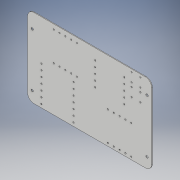
# Autodesk Inventor part: circuit board correct
Saved by Autodesk Inventor 2017 (Build 210142000, 142)
## iProperties
Created: 2017-06-14
Part Number: circuit board correct
Material: Generic
Document SubType Name: Modeling
Designer: slong
Density: 1 g/cm^3
Appearance: Default
Author: slong
Autodesk Inventor part; units mm, degrees
(part 1 of 2)
ref_plane "YZ Plane" through (0, 0, 0) normal (1, 0, 0) x (0, 1, 0)
ref_plane "XZ Plane" through (0, 0, 0) normal (0, 1, 0) x (-1, 0, 0)
ref_plane "XY Plane" through (0, 0, 0) normal (0, 0, 1) x (1, 0, 0)
sketch "Sketch1" plane through (0, 0, 0) normal (0, 0, 1) x (1, 0, 0)
  line L0 (17.0785, 215.8869) -> (322.9005, 215.8869)
  spline S0 degree 3 poles (322.9005, 215.8869) (332.3255, 215.8869) (339.9659, 208.2464) (339.9659, 198.8215) knots 1 1 1 1 2 2 2 2
  line L1 (322.9005, 215.8869) -> (332.3255, 215.8869) construction
  line L2 (332.3255, 215.8869) -> (339.9659, 208.2464) construction
  line L3 (339.9659, 208.2464) -> (339.9659, 198.8215) construction
  line L4 (339.9659, 198.8215) -> (339.9659, 17.0785)
  spline S1 degree 3 poles (339.9659, 17.0785) (339.9659, 7.6536) (332.3255, 0.0131) (322.9005, 0.0131) knots 3 3 3 3 4 4 4 4
  line L5 (339.9659, 17.0785) -> (339.9659, 7.6536) construction
  line L6 (339.9659, 7.6536) -> (332.3255, 0.0131) construction
  line L7 (332.3255, 0.0131) -> (322.9005, 0.0131) construction
  line L8 (322.9005, 0.0131) -> (17.0785, 0.0131)
  spline S2 degree 3 poles (17.0785, 0.0131) (7.6536, 0.0131) (0.0131, 7.6536) (0.0131, 17.0785) knots 5 5 5 5 6 6 6 6
  line L9 (17.0785, 0.0131) -> (7.6536, 0.0131) construction
  line L10 (7.6536, 0.0131) -> (0.0131, 7.6536) construction
  line L11 (0.0131, 7.6536) -> (0.0131, 17.0785) construction
  line L12 (0.0131, 17.0785) -> (0.0131, 198.8215)
  spline S3 degree 3 poles (0.0131, 198.8215) (0.0131, 208.2464) (7.6536, 215.8869) (17.0785, 215.8869) knots 7 7 7 7 8 8 8 8
  line L13 (0.0131, 198.8215) -> (0.0131, 208.2464) construction
  line L14 (0.0131, 208.2464) -> (7.6536, 215.8869) construction
  line L15 (7.6536, 215.8869) -> (17.0785, 215.8869) construction
  spline S4 degree 3 poles (12.7, 177.7884) (14.4471, 177.7884) (15.8634, 176.3721) (15.8634, 174.625) (15.8634, 172.8779) (14.4471, 171.4616) (12.7, 171.4616) (10.9529, 171.4616) (9.5366, 172.8779) (9.5366, 174.625) (9.5366, 176.3721) (10.9529, 177.7884) (12.7, 177.7884) knots 0 0 0 0 1 1 1 2 2 2 3 3 3 4 4 4 4
  line L16 (12.7, 177.7884) -> (14.4471, 177.7884) construction
  line L17 (14.4471, 177.7884) -> (15.8634, 176.3721) construction
  line L18 (15.8634, 176.3721) -> (15.8634, 174.625) construction
  line L19 (15.8634, 174.625) -> (15.8634, 172.8779) construction
  line L20 (15.8634, 172.8779) -> (14.4471, 171.4616) construction
  line L21 (14.4471, 171.4616) -> (12.7, 171.4616) construction
  line L22 (12.7, 171.4616) -> (10.9529, 171.4616) construction
  line L23 (10.9529, 171.4616) -> (9.5366, 172.8779) construction
  line L24 (9.5366, 172.8779) -> (9.5366, 174.625) construction
  line L25 (9.5366, 174.625) -> (9.5366, 176.3721) construction
  line L26 (9.5366, 176.3721) -> (10.9529, 177.7884) construction
  line L27 (10.9529, 177.7884) -> (12.7, 177.7884) construction
  spline S5 degree 3 poles (12.7, 31.7384) (14.4471, 31.7384) (15.8634, 30.3221) (15.8634, 28.575) (15.8634, 26.8279) (14.4471, 25.4116) (12.7, 25.4116) (10.9529, 25.4116) (9.5366, 26.8279) (9.5366, 28.575) (9.5366, 30.3221) (10.9529, 31.7384) (12.7, 31.7384) knots 0 0 0 0 1 1 1 2 2 2 3 3 3 4 4 4 4
  line L28 (12.7, 31.7384) -> (14.4471, 31.7384) construction
  line L29 (14.4471, 31.7384) -> (15.8634, 30.3221) construction
  line L30 (15.8634, 30.3221) -> (15.8634, 28.575) construction
  line L31 (15.8634, 28.575) -> (15.8634, 26.8279) construction
  line L32 (15.8634, 26.8279) -> (14.4471, 25.4116) construction
  line L33 (14.4471, 25.4116) -> (12.7, 25.4116) construction
  line L34 (12.7, 25.4116) -> (10.9529, 25.4116) construction
  line L35 (10.9529, 25.4116) -> (9.5366, 26.8279) construction
  line L36 (9.5366, 26.8279) -> (9.5366, 28.575) construction
  line L37 (9.5366, 28.575) -> (9.5366, 30.3221) construction
  line L38 (9.5366, 30.3221) -> (10.9529, 31.7384) construction
  line L39 (10.9529, 31.7384) -> (12.7, 31.7384) construction
  spline S6 degree 3 poles (327.279, 177.7884) (329.0261, 177.7884) (330.4424, 176.3721) (330.4424, 174.625) (330.4424, 172.8779) (329.0261, 171.4616) (327.279, 171.4616) (325.5319, 171.4616) (324.1156, 172.8779) (324.1156, 174.625) (324.1156, 176.3721) (325.5319, 177.7884) (327.279, 177.7884) knots 0 0 0 0 1 1 1 2 2 2 3 3 3 4 4 4 4
  line L40 (327.279, 177.7884) -> (329.0261, 177.7884) construction
  line L41 (329.0261, 177.7884) -> (330.4424, 176.3721) construction
  line L42 (330.4424, 176.3721) -> (330.4424, 174.625) construction
  line L43 (330.4424, 174.625) -> (330.4424, 172.8779) construction
  line L44 (330.4424, 172.8779) -> (329.0261, 171.4616) construction
  line L45 (329.0261, 171.4616) -> (327.279, 171.4616) construction
  line L46 (327.279, 171.4616) -> (325.5319, 171.4616) construction
  line L47 (325.5319, 171.4616) -> (324.1156, 172.8779) construction
  line L48 (324.1156, 172.8779) -> (324.1156, 174.625) construction
  line L49 (324.1156, 174.625) -> (324.1156, 176.3721) construction
  line L50 (324.1156, 176.3721) -> (325.5319, 177.7884) construction
  line L51 (325.5319, 177.7884) -> (327.279, 177.7884) construction
  spline S7 degree 3 poles (327.279, 31.7384) (329.0261, 31.7384) (330.4424, 30.3221) (330.4424, 28.575) (330.4424, 26.8279) (329.0261, 25.4116) (327.279, 25.4116) (325.5319, 25.4116) (324.1156, 26.8279) (324.1156, 28.575) (324.1156, 30.3221) (325.5319, 31.7384) (327.279, 31.7384) knots 0 0 0 0 1 1 1 2 2 2 3 3 3 4 4 4 4
  line L52 (327.279, 31.7384) -> (329.0261, 31.7384) construction
  line L53 (329.0261, 31.7384) -> (330.4424, 30.3221) construction
  line L54 (330.4424, 30.3221) -> (330.4424, 28.575) construction
  line L55 (330.4424, 28.575) -> (330.4424, 26.8279) construction
  line L56 (330.4424, 26.8279) -> (329.0261, 25.4116) construction
  line L57 (329.0261, 25.4116) -> (327.279, 25.4116) construction
  line L58 (327.279, 25.4116) -> (325.5319, 25.4116) construction
  line L59 (325.5319, 25.4116) -> (324.1156, 26.8279) construction
  line L60 (324.1156, 26.8279) -> (324.1156, 28.575) construction
  line L61 (324.1156, 28.575) -> (324.1156, 30.3221) construction
  line L62 (324.1156, 30.3221) -> (325.5319, 31.7384) construction
  line L63 (325.5319, 31.7384) -> (327.279, 31.7384) construction
  spline S8 degree 3 poles (310.8612, 184.086) (310.8612, 183.106) (310.0414, 182.3108) (309.0314, 182.3108) (308.0224, 182.3108) (307.2012, 183.106) (307.2012, 184.086) (307.2012, 185.0656) (308.0224, 185.8608) (309.0314, 185.8608) (310.0414, 185.8608) (310.8612, 185.0656) (310.8612, 184.086) knots 0 0 0 0 1 1 1 2 2 2 3 3 3 4 4 4 4
  line L64 (310.8612, 184.086) -> (310.8612, 183.106) construction
  line L65 (310.8612, 183.106) -> (310.0414, 182.3108) construction
  line L66 (310.0414, 182.3108) -> (309.0314, 182.3108) construction
  line L67 (309.0314, 182.3108) -> (308.0224, 182.3108) construction
  line L68 (308.0224, 182.3108) -> (307.2012, 183.106) construction
  line L69 (307.2012, 183.106) -> (307.2012, 184.086) construction
  line L70 (307.2012, 184.086) -> (307.2012, 185.0656) construction
  line L71 (307.2012, 185.0656) -> (308.0224, 185.8608) construction
  line L72 (308.0224, 185.8608) -> (309.0314, 185.8608) construction
  line L73 (309.0314, 185.8608) -> (310.0414, 185.8608) construction
  line L74 (310.0414, 185.8608) -> (310.8612, 185.0656) construction
  line L75 (310.8612, 185.0656) -> (310.8612, 184.086) construction
  spline S9 degree 3 poles (286.8614, 184.28) (286.8614, 183.2852) (286.0415, 182.4777) (285.0312, 182.4777) (284.0212, 182.4777) (283.2013, 183.2852) (283.2013, 184.28) (283.2013, 185.2752) (284.0212, 186.0827) (285.0312, 186.0827) (286.0415, 186.0827) (286.8614, 185.2752) (286.8614, 184.28) knots 0 0 0 0 1 1 1 2 2 2 3 3 3 4 4 4 4
  line L76 (286.8614, 184.28) -> (286.8614, 183.2852) construction
  line L77 (286.8614, 183.2852) -> (286.0415, 182.4777) construction
  line L78 (286.0415, 182.4777) -> (285.0312, 182.4777) construction
  line L79 (285.0312, 182.4777) -> (284.0212, 182.4777) construction
  line L80 (284.0212, 182.4777) -> (283.2013, 183.2852) construction
  line L81 (283.2013, 183.2852) -> (283.2013, 184.28) construction
  line L82 (283.2013, 184.28) -> (283.2013, 185.2752) construction
  line L83 (283.2013, 185.2752) -> (284.0212, 186.0827) construction
  line L84 (284.0212, 186.0827) -> (285.0312, 186.0827) construction
  line L85 (285.0312, 186.0827) -> (286.0415, 186.0827) construction
  line L86 (286.0415, 186.0827) -> (286.8614, 185.2752) construction
  line L87 (286.8614, 185.2752) -> (286.8614, 184.28) construction
  spline S10 degree 3 poles (310.8612, 207.9729) (310.8612, 206.9929) (310.0414, 206.1977) (309.0314, 206.1977) (308.0224, 206.1977) (307.2012, 206.9929) (307.2012, 207.9729) (307.2012, 208.9526) (308.0224, 209.7492) (309.0314, 209.7492) (310.0414, 209.7492) (310.8612, 208.9526) (310.8612, 207.9729) knots 0 0 0 0 1 1 1 2 2 2 3 3 3 4 4 4 4
  line L88 (310.8612, 207.9729) -> (310.8612, 206.9929) construction
  line L89 (310.8612, 206.9929) -> (310.0414, 206.1977) construction
  line L90 (310.0414, 206.1977) -> (309.0314, 206.1977) construction
  line L91 (309.0314, 206.1977) -> (308.0224, 206.1977) construction
  line L92 (308.0224, 206.1977) -> (307.2012, 206.9929) construction
  line L93 (307.2012, 206.9929) -> (307.2012, 207.9729) construction
  line L94 (307.2012, 207.9729) -> (307.2012, 208.9526) construction
  line L95 (307.2012, 208.9526) -> (308.0224, 209.7492) construction
  line L96 (308.0224, 209.7492) -> (309.0314, 209.7492) construction
  line L97 (309.0314, 209.7492) -> (310.0414, 209.7492) construction
  line L98 (310.0414, 209.7492) -> (310.8612, 208.9526) construction
  line L99 (310.8612, 208.9526) -> (310.8612, 207.9729) construction
  spline S11 degree 3 poles (286.8614, 208.1683) (286.8614, 207.1735) (286.0415, 206.366) (285.0312, 206.366) (284.0212, 206.366) (283.2013, 207.1735) (283.2013, 208.1683) (283.2013, 209.1635) (284.0212, 209.9711) (285.0312, 209.9711) (286.0415, 209.9711) (286.8614, 209.1635) (286.8614, 208.1683) knots 0 0 0 0 1 1 1 2 2 2 3 3 3 4 4 4 4
  line L100 (286.8614, 208.1683) -> (286.8614, 207.1735) construction
  line L101 (286.8614, 207.1735) -> (286.0415, 206.366) construction
  line L102 (286.0415, 206.366) -> (285.0312, 206.366) construction
  line L103 (285.0312, 206.366) -> (284.0212, 206.366) construction
  line L104 (284.0212, 206.366) -> (283.2013, 207.1735) construction
  line L105 (283.2013, 207.1735) -> (283.2013, 208.1683) construction
  line L106 (283.2013, 208.1683) -> (283.2013, 209.1635) construction
  line L107 (283.2013, 209.1635) -> (284.0212, 209.9711) construction
  line L108 (284.0212, 209.9711) -> (285.0312, 209.9711) construction
  line L109 (285.0312, 209.9711) -> (286.0415, 209.9711) construction
  line L110 (286.0415, 209.9711) -> (286.8614, 209.1635) construction
  line L111 (286.8614, 209.1635) -> (286.8614, 208.1683) construction
  spline S12 degree 3 poles (310.8612, 148.7399) (310.8612, 147.7599) (310.0414, 146.9647) (309.0314, 146.9647) (308.0224, 146.9647) (307.2012, 147.7599) (307.2012, 148.7399) (307.2012, 149.7196) (308.0224, 150.5147) (309.0314, 150.5147) (310.0414, 150.5147) (310.8612, 149.7196) (310.8612, 148.7399) knots 0 0 0 0 1 1 1 2 2 2 3 3 3 4 4 4 4
  line L112 (310.8612, 148.7399) -> (310.8612, 147.7599) construction
  line L113 (310.8612, 147.7599) -> (310.0414, 146.9647) construction
  line L114 (310.0414, 146.9647) -> (309.0314, 146.9647) construction
  line L115 (309.0314, 146.9647) -> (308.0224, 146.9647) construction
  line L116 (308.0224, 146.9647) -> (307.2012, 147.7599) construction
  line L117 (307.2012, 147.7599) -> (307.2012, 148.7399) construction
  line L118 (307.2012, 148.7399) -> (307.2012, 149.7196) construction
  line L119 (307.2012, 149.7196) -> (308.0224, 150.5147) construction
  line L120 (308.0224, 150.5147) -> (309.0314, 150.5147) construction
  line L121 (309.0314, 150.5147) -> (310.0414, 150.5147) construction
  line L122 (310.0414, 150.5147) -> (310.8612, 149.7196) construction
  line L123 (310.8612, 149.7196) -> (310.8612, 148.7399) construction
  spline S13 degree 3 poles (286.8614, 148.9339) (286.8614, 147.9391) (286.0415, 147.1316) (285.0312, 147.1316) (284.0212, 147.1316) (283.2013, 147.9391) (283.2013, 148.9339) (283.2013, 149.9291) (284.0212, 150.7366) (285.0312, 150.7366) (286.0415, 150.7366) (286.8614, 149.9291) (286.8614, 148.9339) knots 0 0 0 0 1 1 1 2 2 2 3 3 3 4 4 4 4
  line L124 (286.8614, 148.9339) -> (286.8614, 147.9391) construction
  line L125 (286.8614, 147.9391) -> (286.0415, 147.1316) construction
  line L126 (286.0415, 147.1316) -> (285.0312, 147.1316) construction
  line L127 (285.0312, 147.1316) -> (284.0212, 147.1316) construction
  line L128 (284.0212, 147.1316) -> (283.2013, 147.9391) construction
  line L129 (283.2013, 147.9391) -> (283.2013, 148.9339) construction
  line L130 (283.2013, 148.9339) -> (283.2013, 149.9291) construction
  line L131 (283.2013, 149.9291) -> (284.0212, 150.7366) construction
  line L132 (284.0212, 150.7366) -> (285.0312, 150.7366) construction
  line L133 (285.0312, 150.7366) -> (286.0415, 150.7366) construction
  line L134 (286.0415, 150.7366) -> (286.8614, 149.9291) construction
  line L135 (286.8614, 149.9291) -> (286.8614, 148.9339) construction
  spline S14 degree 3 poles (310.8612, 172.6269) (310.8612, 171.6469) (310.0414, 170.8517) (309.0314, 170.8517) (308.0224, 170.8517) (307.2012, 171.6469) (307.2012, 172.6269) (307.2012, 173.6065) (308.0224, 174.4031) (309.0314, 174.4031) (310.0414, 174.4031) (310.8612, 173.6065) (310.8612, 172.6269) knots 0 0 0 0 1 1 1 2 2 2 3 3 3 4 4 4 4
  line L136 (310.8612, 172.6269) -> (310.8612, 171.6469) construction
  line L137 (310.8612, 171.6469) -> (310.0414, 170.8517) construction
  line L138 (310.0414, 170.8517) -> (309.0314, 170.8517) construction
  line L139 (309.0314, 170.8517) -> (308.0224, 170.8517) construction
  line L140 (308.0224, 170.8517) -> (307.2012, 171.6469) construction
  line L141 (307.2012, 171.6469) -> (307.2012, 172.6269) construction
  line L142 (307.2012, 172.6269) -> (307.2012, 173.6065) construction
  line L143 (307.2012, 173.6065) -> (308.0224, 174.4031) construction
  line L144 (308.0224, 174.4031) -> (309.0314, 174.4031) construction
  line L145 (309.0314, 174.4031) -> (310.0414, 174.4031) construction
  line L146 (310.0414, 174.4031) -> (310.8612, 173.6065) construction
  line L147 (310.8612, 173.6065) -> (310.8612, 172.6269) construction
  spline S15 degree 3 poles (286.8614, 172.8223) (286.8614, 171.8274) (286.0415, 171.0199) (285.0312, 171.0199) (284.0212, 171.0199) (283.2013, 171.8274) (283.2013, 172.8223) (283.2013, 173.8175) (284.0212, 174.625) (285.0312, 174.625) (286.0415, 174.625) (286.8614, 173.8175) (286.8614, 172.8223) knots 0 0 0 0 1 1 1 2 2 2 3 3 3 4 4 4 4
  line L148 (286.8614, 172.8223) -> (286.8614, 171.8274) construction
  line L149 (286.8614, 171.8274) -> (286.0415, 171.0199) construction
  line L150 (286.0415, 171.0199) -> (285.0312, 171.0199) construction
  line L151 (285.0312, 171.0199) -> (284.0212, 171.0199) construction
  line L152 (284.0212, 171.0199) -> (283.2013, 171.8274) construction
  line L153 (283.2013, 171.8274) -> (283.2013, 172.8223) construction
  line L154 (283.2013, 172.8223) -> (283.2013, 173.8175) construction
  line L155 (283.2013, 173.8175) -> (284.0212, 174.625) construction
  line L156 (284.0212, 174.625) -> (285.0312, 174.625) construction
  line L157 (285.0312, 174.625) -> (286.0415, 174.625) construction
  line L158 (286.0415, 174.625) -> (286.8614, 173.8175) construction
  line L159 (286.8614, 173.8175) -> (286.8614, 172.8223) construction
  spline S16 degree 3 poles (73.3234, 122.6835) (73.3234, 121.6731) (72.5036, 120.8533) (71.4936, 120.8533) (70.4832, 120.8533) (69.6634, 121.6731) (69.6634, 122.6835) (69.6634, 123.6935) (70.4832, 124.5134) (71.4936, 124.5134) (72.5036, 124.5134) (73.3234, 123.6935) (73.3234, 122.6835) knots 0 0 0 0 1 1 1 2 2 2 3 3 3 4 4 4 4
  line L160 (73.3234, 122.6835) -> (73.3234, 121.6731) construction
  line L161 (73.3234, 121.6731) -> (72.5036, 120.8533) construction
  line L162 (72.5036, 120.8533) -> (71.4936, 120.8533) construction
  line L163 (71.4936, 120.8533) -> (70.4832, 120.8533) construction
  line L164 (70.4832, 120.8533) -> (69.6634, 121.6731) construction
  line L165 (69.6634, 121.6731) -> (69.6634, 122.6835) construction
  line L166 (69.6634, 122.6835) -> (69.6634, 123.6935) construction
  line L167 (69.6634, 123.6935) -> (70.4832, 124.5134) construction
  line L168 (70.4832, 124.5134) -> (71.4936, 124.5134) construction
  line L169 (71.4936, 124.5134) -> (72.5036, 124.5134) construction
  line L170 (72.5036, 124.5134) -> (73.3234, 123.6935) construction
  line L171 (73.3234, 123.6935) -> (73.3234, 122.6835) construction
  spline S17 degree 3 poles (89.324, 122.6835) (89.324, 121.6731) (88.5038, 120.8533) (87.4938, 120.8533) (86.4838, 120.8533) (85.6639, 121.6731) (85.6639, 122.6835) (85.6639, 123.6935) (86.4838, 124.5134) (87.4938, 124.5134) (88.5038, 124.5134) (89.324, 123.6935) (89.324, 122.6835) knots 0 0 0 0 1 1 1 2 2 2 3 3 3 4 4 4 4
  line L172 (89.324, 122.6835) -> (89.324, 121.6731) construction
  line L173 (89.324, 121.6731) -> (88.5038, 120.8533) construction
  line L174 (88.5038, 120.8533) -> (87.4938, 120.8533) construction
  line L175 (87.4938, 120.8533) -> (86.4838, 120.8533) construction
  line L176 (86.4838, 120.8533) -> (85.6639, 121.6731) construction
  line L177 (85.6639, 121.6731) -> (85.6639, 122.6835) construction
  line L178 (85.6639, 122.6835) -> (85.6639, 123.6935) construction
  line L179 (85.6639, 123.6935) -> (86.4838, 124.5134) construction
  line L180 (86.4838, 124.5134) -> (87.4938, 124.5134) construction
  line L181 (87.4938, 124.5134) -> (88.5038, 124.5134) construction
  line L182 (88.5038, 124.5134) -> (89.324, 123.6935) construction
  line L183 (89.324, 123.6935) -> (89.324, 122.6835) construction
  spline S18 degree 3 poles (101.6656, 122.62) (101.6656, 121.6153) (102.4854, 120.7997) (103.4955, 120.7997) (104.5058, 120.7997) (105.3257, 121.6153) (105.3257, 122.62) (105.3257, 123.6247) (104.5058, 124.4417) (103.4955, 124.4417) (102.4854, 124.4417) (101.6656, 123.6247) (101.6656, 122.62) knots 0 0 0 0 1 1 1 2 2 2 3 3 3 4 4 4 4
  line L184 (101.6656, 122.62) -> (101.6656, 121.6153) construction
  line L185 (101.6656, 121.6153) -> (102.4854, 120.7997) construction
  line L186 (102.4854, 120.7997) -> (103.4955, 120.7997) construction
  line L187 (103.4955, 120.7997) -> (104.5058, 120.7997) construction
  line L188 (104.5058, 120.7997) -> (105.3257, 121.6153) construction
  line L189 (105.3257, 121.6153) -> (105.3257, 122.62) construction
  line L190 (105.3257, 122.62) -> (105.3257, 123.6247) construction
  line L191 (105.3257, 123.6247) -> (104.5058, 124.4417) construction
  line L192 (104.5058, 124.4417) -> (103.4955, 124.4417) construction
  line L193 (103.4955, 124.4417) -> (102.4854, 124.4417) construction
  line L194 (102.4854, 124.4417) -> (101.6656, 123.6247) construction
  line L195 (101.6656, 123.6247) -> (101.6656, 122.62) construction
  spline S19 degree 3 poles (121.3259, 122.62) (121.3259, 121.6153) (120.506, 120.7997) (119.496, 120.7997) (118.486, 120.7997) (117.6658, 121.6153) (117.6658, 122.62) (117.6658, 123.6247) (118.486, 124.4417) (119.496, 124.4417) (120.506, 124.4417) (121.3259, 123.6247) (121.3259, 122.62) knots 0 0 0 0 1 1 1 2 2 2 3 3 3 4 4 4 4
  line L196 (121.3259, 122.62) -> (121.3259, 121.6153) construction
  line L197 (121.3259, 121.6153) -> (120.506, 120.7997) construction
  line L198 (120.506, 120.7997) -> (119.496, 120.7997) construction
  line L199 (119.496, 120.7997) -> (118.486, 120.7997) construction
  line L200 (118.486, 120.7997) -> (117.6658, 121.6153) construction
  line L201 (117.6658, 121.6153) -> (117.6658, 122.62) construction
  line L202 (117.6658, 122.62) -> (117.6658, 123.6247) construction
  line L203 (117.6658, 123.6247) -> (118.486, 124.4417) construction
  line L204 (118.486, 124.4417) -> (119.496, 124.4417) construction
  line L205 (119.496, 124.4417) -> (120.506, 124.4417) construction
  line L206 (120.506, 124.4417) -> (121.3259, 123.6247) construction
  line L207 (121.3259, 123.6247) -> (121.3259, 122.62) construction
  spline S20 degree 3 poles (137.3265, 122.4905) (137.3265, 121.4953) (136.5052, 120.6878) (135.4963, 120.6878) (134.4863, 120.6878) (133.6664, 121.4953) (133.6664, 122.4905) (133.6664, 123.4854) (134.4863, 124.2929) (135.4963, 124.2929) (136.5052, 124.2929) (137.3265, 123.4854) (137.3265, 122.4905) knots 0 0 0 0 1 1 1 2 2 2 3 3 3 4 4 4 4
  line L208 (137.3265, 122.4905) -> (137.3265, 121.4953) construction
  line L209 (137.3265, 121.4953) -> (136.5052, 120.6878) construction
  line L210 (136.5052, 120.6878) -> (135.4963, 120.6878) construction
  line L211 (135.4963, 120.6878) -> (134.4863, 120.6878) construction
  line L212 (134.4863, 120.6878) -> (133.6664, 121.4953) construction
  line L213 (133.6664, 121.4953) -> (133.6664, 122.4905) construction
  line L214 (133.6664, 122.4905) -> (133.6664, 123.4854) construction
  line L215 (133.6664, 123.4854) -> (134.4863, 124.2929) construction
  line L216 (134.4863, 124.2929) -> (135.4963, 124.2929) construction
  line L217 (135.4963, 124.2929) -> (136.5052, 124.2929) construction
  line L218 (136.5052, 124.2929) -> (137.3265, 123.4854) construction
  line L219 (137.3265, 123.4854) -> (137.3265, 122.4905) construction
  spline S21 degree 3 poles (73.3236, 202.6826) (73.3236, 201.6726) (72.5034, 200.8527) (71.4934, 200.8527) (70.4834, 200.8527) (69.6636, 201.6726) (69.6636, 202.6826) (69.6636, 203.6926) (70.4834, 204.5128) (71.4934, 204.5128) (72.5034, 204.5128) (73.3236, 203.6926) (73.3236, 202.6826) knots 0 0 0 0 1 1 1 2 2 2 3 3 3 4 4 4 4
  line L220 (73.3236, 202.6826) -> (73.3236, 201.6726) construction
  line L221 (73.3236, 201.6726) -> (72.5034, 200.8527) construction
  line L222 (72.5034, 200.8527) -> (71.4934, 200.8527) construction
  line L223 (71.4934, 200.8527) -> (70.4834, 200.8527) construction
  line L224 (70.4834, 200.8527) -> (69.6636, 201.6726) construction
  line L225 (69.6636, 201.6726) -> (69.6636, 202.6826) construction
  line L226 (69.6636, 202.6826) -> (69.6636, 203.6926) construction
  line L227 (69.6636, 203.6926) -> (70.4834, 204.5128) construction
  line L228 (70.4834, 204.5128) -> (71.4934, 204.5128) construction
  line L229 (71.4934, 204.5128) -> (72.5034, 204.5128) construction
  line L230 (72.5034, 204.5128) -> (73.3236, 203.6926) construction
  line L231 (73.3236, 203.6926) -> (73.3236, 202.6826) construction
  spline S22 degree 3 poles (89.3238, 202.6826) (89.3238, 201.6726) (88.504, 200.8527) (87.494, 200.8527) (86.4836, 200.8527) (85.6638, 201.6726) (85.6638, 202.6826) (85.6638, 203.6926) (86.4836, 204.5128) (87.494, 204.5128) (88.504, 204.5128) (89.3238, 203.6926) (89.3238, 202.6826) knots 0 0 0 0 1 1 1 2 2 2 3 3 3 4 4 4 4
  line L232 (89.3238, 202.6826) -> (89.3238, 201.6726) construction
  line L233 (89.3238, 201.6726) -> (88.504, 200.8527) construction
  line L234 (88.504, 200.8527) -> (87.494, 200.8527) construction
  line L235 (87.494, 200.8527) -> (86.4836, 200.8527) construction
  line L236 (86.4836, 200.8527) -> (85.6638, 201.6726) construction
  line L237 (85.6638, 201.6726) -> (85.6638, 202.6826) construction
  line L238 (85.6638, 202.6826) -> (85.6638, 203.6926) construction
  line L239 (85.6638, 203.6926) -> (86.4836, 204.5128) construction
  line L240 (86.4836, 204.5128) -> (87.494, 204.5128) construction
  line L241 (87.494, 204.5128) -> (88.504, 204.5128) construction
  line L242 (88.504, 204.5128) -> (89.3238, 203.6926) construction
  line L243 (89.3238, 203.6926) -> (89.3238, 202.6826) construction
  spline S23 degree 3 poles (105.3258, 202.6191) (105.3258, 201.6147) (104.5056, 200.7987) (103.4956, 200.7987) (102.4856, 200.7987) (101.6658, 201.6147) (101.6658, 202.6191) (101.6658, 203.6252) (102.4856, 204.4412) (103.4956, 204.4412) (104.5056, 204.4412) (105.3258, 203.6252) (105.3258, 202.6191) knots 0 0 0 0 1 1 1 2 2 2 3 3 3 4 4 4 4
  line L244 (105.3258, 202.6191) -> (105.3258, 201.6147) construction
  line L245 (105.3258, 201.6147) -> (104.5056, 200.7987) construction
  line L246 (104.5056, 200.7987) -> (103.4956, 200.7987) construction
  line L247 (103.4956, 200.7987) -> (102.4856, 200.7987) construction
  line L248 (102.4856, 200.7987) -> (101.6658, 201.6147) construction
  line L249 (101.6658, 201.6147) -> (101.6658, 202.6191) construction
  line L250 (101.6658, 202.6191) -> (101.6658, 203.6252) construction
  line L251 (101.6658, 203.6252) -> (102.4856, 204.4412) construction
  line L252 (102.4856, 204.4412) -> (103.4956, 204.4412) construction
  line L253 (103.4956, 204.4412) -> (104.5056, 204.4412) construction
  line L254 (104.5056, 204.4412) -> (105.3258, 203.6252) construction
  line L255 (105.3258, 203.6252) -> (105.3258, 202.6191) construction
  spline S24 degree 3 poles (121.326, 202.6191) (121.326, 201.6147) (120.5062, 200.7987) (119.4962, 200.7987) (118.4858, 200.7987) (117.6659, 201.6147) (117.6659, 202.6191) (117.6659, 203.6252) (118.4858, 204.4412) (119.4962, 204.4412) (120.5062, 204.4412) (121.326, 203.6252) (121.326, 202.6191) knots 0 0 0 0 1 1 1 2 2 2 3 3 3 4 4 4 4
  line L256 (121.326, 202.6191) -> (121.326, 201.6147) construction
  line L257 (121.326, 201.6147) -> (120.5062, 200.7987) construction
  line L258 (120.5062, 200.7987) -> (119.4962, 200.7987) construction
  line L259 (119.4962, 200.7987) -> (118.4858, 200.7987) construction
  line L260 (118.4858, 200.7987) -> (117.6659, 201.6147) construction
  line L261 (117.6659, 201.6147) -> (117.6659, 202.6191) construction
  line L262 (117.6659, 202.6191) -> (117.6659, 203.6252) construction
  line L263 (117.6659, 203.6252) -> (118.4858, 204.4412) construction
  line L264 (118.4858, 204.4412) -> (119.4962, 204.4412) construction
  line L265 (119.4962, 204.4412) -> (120.5062, 204.4412) construction
  line L266 (120.5062, 204.4412) -> (121.326, 203.6252) construction
  line L267 (121.326, 203.6252) -> (121.326, 202.6191) construction
  spline S25 degree 3 poles (137.3252, 202.4896) (137.3252, 201.4948) (136.5053, 200.6872) (135.495, 200.6872) (134.4864, 200.6872) (133.6665, 201.4948) (133.6665, 202.4896) (133.6665, 203.4848) (134.4864, 204.2923) (135.495, 204.2923) (136.5053, 204.2923) (137.3252, 203.4848) (137.3252, 202.4896) knots 0 0 0 0 1 1 1 2 2 2 3 3 3 4 4 4 4
  line L268 (137.3252, 202.4896) -> (137.3252, 201.4948) construction
  line L269 (137.3252, 201.4948) -> (136.5053, 200.6872) construction
  line L270 (136.5053, 200.6872) -> (135.495, 200.6872) construction
  line L271 (135.495, 200.6872) -> (134.4864, 200.6872) construction
  line L272 (134.4864, 200.6872) -> (133.6665, 201.4948) construction
  line L273 (133.6665, 201.4948) -> (133.6665, 202.4896) construction
  line L274 (133.6665, 202.4896) -> (133.6665, 203.4848) construction
  line L275 (133.6665, 203.4848) -> (134.4864, 204.2923) construction
  line L276 (134.4864, 204.2923) -> (135.495, 204.2923) construction
  line L277 (135.495, 204.2923) -> (136.5053, 204.2923) construction
  line L278 (136.5053, 204.2923) -> (137.3252, 203.4848) construction
  line L279 (137.3252, 203.4848) -> (137.3252, 202.4896) construction
  spline S26 degree 3 poles (126.1694, 103.4986) (125.1594, 103.4986) (124.3396, 104.3184) (124.3396, 105.3288) (124.3396, 106.3388) (125.1594, 107.1586) (126.1694, 107.1586) (127.1798, 107.1586) (127.9996, 106.3388) (127.9996, 105.3288) (127.9996, 104.3184) (127.1798, 103.4986) (126.1694, 103.4986) knots 0 0 0 0 1 1 1 2 2 2 3 3 3 4 4 4 4
  line L280 (126.1694, 103.4986) -> (125.1594, 103.4986) construction
  line L281 (125.1594, 103.4986) -> (124.3396, 104.3184) construction
  line L282 (124.3396, 104.3184) -> (124.3396, 105.3288) construction
  line L283 (124.3396, 105.3288) -> (124.3396, 106.3388) construction
  line L284 (124.3396, 106.3388) -> (125.1594, 107.1586) construction
  line L285 (125.1594, 107.1586) -> (126.1694, 107.1586) construction
  line L286 (126.1694, 107.1586) -> (127.1798, 107.1586) construction
  line L287 (127.1798, 107.1586) -> (127.9996, 106.3388) construction
  line L288 (127.9996, 106.3388) -> (127.9996, 105.3288) construction
  line L289 (127.9996, 105.3288) -> (127.9996, 104.3184) construction
  line L290 (127.9996, 104.3184) -> (127.1798, 103.4986) construction
  line L291 (127.1798, 103.4986) -> (126.1694, 103.4986) construction
  spline S27 degree 3 poles (126.1694, 87.4997) (125.1594, 87.4997) (124.3396, 88.3196) (124.3396, 89.3282) (124.3396, 90.3382) (125.1594, 91.1584) (126.1694, 91.1584) (127.1798, 91.1584) (127.9996, 90.3382) (127.9996, 89.3282) (127.9996, 88.3196) (127.1798, 87.4997) (126.1694, 87.4997) knots 0 0 0 0 1 1 1 2 2 2 3 3 3 4 4 4 4
  line L292 (126.1694, 87.4997) -> (125.1594, 87.4997) construction
  line L293 (125.1594, 87.4997) -> (124.3396, 88.3196) construction
  line L294 (124.3396, 88.3196) -> (124.3396, 89.3282) construction
  line L295 (124.3396, 89.3282) -> (124.3396, 90.3382) construction
  line L296 (124.3396, 90.3382) -> (125.1594, 91.1584) construction
  line L297 (125.1594, 91.1584) -> (126.1694, 91.1584) construction
  line L298 (126.1694, 91.1584) -> (127.1798, 91.1584) construction
  line L299 (127.1798, 91.1584) -> (127.9996, 90.3382) construction
  line L300 (127.9996, 90.3382) -> (127.9996, 89.3282) construction
  line L301 (127.9996, 89.3282) -> (127.9996, 88.3196) construction
  line L302 (127.9996, 88.3196) -> (127.1798, 87.4997) construction
  line L303 (127.1798, 87.4997) -> (126.1694, 87.4997) construction
  spline S28 degree 3 poles (126.1063, 71.4963) (125.1016, 71.4963) (124.286, 72.3165) (124.286, 73.3265) (124.286, 74.3365) (125.1016, 75.1564) (126.1063, 75.1564) (127.1106, 75.1564) (127.9266, 74.3365) (127.9266, 73.3265) (127.9266, 72.3165) (127.1107, 71.4963) (126.1063, 71.4963) knots 0 0 0 0 1 1 1 2 2 2 3 3 3 4 4 4 4
  line L304 (126.1063, 71.4963) -> (125.1016, 71.4963) construction
  line L305 (125.1016, 71.4963) -> (124.286, 72.3165) construction
  line L306 (124.286, 72.3165) -> (124.286, 73.3265) construction
  line L307 (124.286, 73.3265) -> (124.286, 74.3365) construction
  line L308 (124.286, 74.3365) -> (125.1016, 75.1564) construction
  line L309 (125.1016, 75.1564) -> (126.1063, 75.1564) construction
  line L310 (126.1063, 75.1564) -> (127.1106, 75.1564) construction
  line L311 (127.1106, 75.1564) -> (127.9266, 74.3365) construction
  line L312 (127.9266, 74.3365) -> (127.9266, 73.3265) construction
  line L313 (127.9266, 73.3265) -> (127.9266, 72.3165) construction
  line L314 (127.9266, 72.3165) -> (127.1107, 71.4963) construction
  line L315 (127.1107, 71.4963) -> (126.1063, 71.4963) construction
  spline S29 degree 3 poles (126.1063, 55.4975) (125.1016, 55.4975) (124.286, 56.3174) (124.286, 57.3274) (124.286, 58.3377) (125.1016, 59.1576) (126.1063, 59.1576) (127.1106, 59.1576) (127.9266, 58.3377) (127.9266, 57.3274) (127.9266, 56.3174) (127.1107, 55.4975) (126.1063, 55.4975) knots 0 0 0 0 1 1 1 2 2 2 3 3 3 4 4 4 4
  line L316 (126.1063, 55.4975) -> (125.1016, 55.4975) construction
  line L317 (125.1016, 55.4975) -> (124.286, 56.3174) construction
  line L318 (124.286, 56.3174) -> (124.286, 57.3274) construction
  line L319 (124.286, 57.3274) -> (124.286, 58.3377) construction
  line L320 (124.286, 58.3377) -> (125.1016, 59.1576) construction
  line L321 (125.1016, 59.1576) -> (126.1063, 59.1576) construction
  line L322 (126.1063, 59.1576) -> (127.1106, 59.1576) construction
  line L323 (127.1106, 59.1576) -> (127.9266, 58.3377) construction
  line L324 (127.9266, 58.3377) -> (127.9266, 57.3274) construction
  line L325 (127.9266, 57.3274) -> (127.9266, 56.3174) construction
  line L326 (127.9266, 56.3174) -> (127.1107, 55.4975) construction
  line L327 (127.1107, 55.4975) -> (126.1063, 55.4975) construction
  spline S30 degree 3 poles (125.9768, 39.4969) (124.9816, 39.4969) (124.1741, 40.3171) (124.1741, 41.3271) (124.1741, 42.3371) (124.9816, 43.157) (125.9768, 43.157) (126.9717, 43.157) (127.7792, 42.3371) (127.7792, 41.3271) (127.7792, 40.3171) (126.9717, 39.4969) (125.9768, 39.4969) knots 0 0 0 0 1 1 1 2 2 2 3 3 3 4 4 4 4
  line L328 (125.9768, 39.4969) -> (124.9816, 39.4969) construction
  line L329 (124.9816, 39.4969) -> (124.1741, 40.3171) construction
  line L330 (124.1741, 40.3171) -> (124.1741, 41.3271) construction
  line L331 (124.1741, 41.3271) -> (124.1741, 42.3371) construction
  line L332 (124.1741, 42.3371) -> (124.9816, 43.157) construction
  line L333 (124.9816, 43.157) -> (125.9768, 43.157) construction
  line L334 (125.9768, 43.157) -> (126.9717, 43.157) construction
  line L335 (126.9717, 43.157) -> (127.7792, 42.3371) construction
  line L336 (127.7792, 42.3371) -> (127.7792, 41.3271) construction
  line L337 (127.7792, 41.3271) -> (127.7792, 40.3171) construction
  line L338 (127.7792, 40.3171) -> (126.9717, 39.4969) construction
  line L339 (126.9717, 39.4969) -> (125.9768, 39.4969) construction
  spline S31 degree 3 poles (125.9768, 23.4967) (124.9816, 23.4967) (124.1741, 24.3165) (124.1741, 25.3265) (124.1741, 26.3369) (124.9816, 27.1567) (125.9768, 27.1567) (126.9717, 27.1567) (127.7792, 26.3369) (127.7792, 25.3265) (127.7792, 24.3165) (126.9717, 23.4967) (125.9768, 23.4967) knots 0 0 0 0 1 1 1 2 2 2 3 3 3 4 4 4 4
  line L340 (125.9768, 23.4967) -> (124.9816, 23.4967) construction
  line L341 (124.9816, 23.4967) -> (124.1741, 24.3165) construction
  line L342 (124.1741, 24.3165) -> (124.1741, 25.3265) construction
  line L343 (124.1741, 25.3265) -> (124.1741, 26.3369) construction
  line L344 (124.1741, 26.3369) -> (124.9816, 27.1567) construction
  line L345 (124.9816, 27.1567) -> (125.9768, 27.1567) construction
  line L346 (125.9768, 27.1567) -> (126.9717, 27.1567) construction
  line L347 (126.9717, 27.1567) -> (127.7792, 26.3369) construction
  line L348 (127.7792, 26.3369) -> (127.7792, 25.3265) construction
  line L349 (127.7792, 25.3265) -> (127.7792, 24.3165) construction
  line L350 (127.7792, 24.3165) -> (126.9717, 23.4967) construction
  line L351 (126.9717, 23.4967) -> (125.9768, 23.4967) construction
  spline S32 degree 3 poles (125.781, 7.4961) (124.8014, 7.4961) (124.0062, 8.3163) (124.0062, 9.3263) (124.0062, 10.3363) (124.8014, 11.1562) (125.781, 11.1562) (126.7607, 11.1562) (127.5573, 10.3363) (127.5573, 9.3263) (127.5573, 8.3163) (126.7607, 7.4961) (125.781, 7.4961) knots 0 0 0 0 1 1 1 2 2 2 3 3 3 4 4 4 4
  line L352 (125.781, 7.4961) -> (124.8014, 7.4961) construction
  line L353 (124.8014, 7.4961) -> (124.0062, 8.3163) construction
  line L354 (124.0062, 8.3163) -> (124.0062, 9.3263) construction
  line L355 (124.0062, 9.3263) -> (124.0062, 10.3363) construction
  line L356 (124.0062, 10.3363) -> (124.8014, 11.1562) construction
  line L357 (124.8014, 11.1562) -> (125.781, 11.1562) construction
  line L358 (125.781, 11.1562) -> (126.7607, 11.1562) construction
  line L359 (126.7607, 11.1562) -> (127.5573, 10.3363) construction
  line L360 (127.5573, 10.3363) -> (127.5573, 9.3263) construction
  line L361 (127.5573, 9.3263) -> (127.5573, 8.3163) construction
  line L362 (127.5573, 8.3163) -> (126.7607, 7.4961) construction
  line L363 (126.7607, 7.4961) -> (125.781, 7.4961) construction
  spline S33 degree 3 poles (38.1694, 103.4986) (37.1594, 103.4986) (36.3395, 104.3184) (36.3395, 105.3288) (36.3395, 106.3388) (37.1594, 107.1586) (38.1694, 107.1586) (39.1794, 107.1586) (39.9996, 106.3388) (39.9996, 105.3288) (39.9996, 104.3184) (39.1794, 103.4986) (38.1694, 103.4986) knots 0 0 0 0 1 1 1 2 2 2 3 3 3 4 4 4 4
  line L364 (38.1694, 103.4986) -> (37.1594, 103.4986) construction
  line L365 (37.1594, 103.4986) -> (36.3395, 104.3184) construction
  line L366 (36.3395, 104.3184) -> (36.3395, 105.3288) construction
  line L367 (36.3395, 105.3288) -> (36.3395, 106.3388) construction
  line L368 (36.3395, 106.3388) -> (37.1594, 107.1586) construction
  line L369 (37.1594, 107.1586) -> (38.1694, 107.1586) construction
  line L370 (38.1694, 107.1586) -> (39.1794, 107.1586) construction
  line L371 (39.1794, 107.1586) -> (39.9996, 106.3388) construction
  line L372 (39.9996, 106.3388) -> (39.9996, 105.3288) construction
  line L373 (39.9996, 105.3288) -> (39.9996, 104.3184) construction
  line L374 (39.9996, 104.3184) -> (39.1794, 103.4986) construction
  line L375 (39.1794, 103.4986) -> (38.1694, 103.4986) construction
  spline S34 degree 3 poles (38.1694, 87.4997) (37.1594, 87.4997) (36.3395, 88.3196) (36.3395, 89.3282) (36.3395, 90.3382) (37.1594, 91.1584) (38.1694, 91.1584) (39.1794, 91.1584) (39.9996, 90.3382) (39.9996, 89.3282) (39.9996, 88.3196) (39.1794, 87.4997) (38.1694, 87.4997) knots 0 0 0 0 1 1 1 2 2 2 3 3 3 4 4 4 4
  line L376 (38.1694, 87.4997) -> (37.1594, 87.4997) construction
  line L377 (37.1594, 87.4997) -> (36.3395, 88.3196) construction
  line L378 (36.3395, 88.3196) -> (36.3395, 89.3282) construction
  line L379 (36.3395, 89.3282) -> (36.3395, 90.3382) construction
  line L380 (36.3395, 90.3382) -> (37.1594, 91.1584) construction
  line L381 (37.1594, 91.1584) -> (38.1694, 91.1584) construction
  line L382 (38.1694, 91.1584) -> (39.1794, 91.1584) construction
  line L383 (39.1794, 91.1584) -> (39.9996, 90.3382) construction
  line L384 (39.9996, 90.3382) -> (39.9996, 89.3282) construction
  line L385 (39.9996, 89.3282) -> (39.9996, 88.3196) construction
  line L386 (39.9996, 88.3196) -> (39.1794, 87.4997) construction
  line L387 (39.1794, 87.4997) -> (38.1694, 87.4997) construction
  spline S35 degree 3 poles (38.1062, 71.4963) (37.1015, 71.4963) (36.2855, 72.3165) (36.2855, 73.3265) (36.2855, 74.3365) (37.1015, 75.1564) (38.1062, 75.1564) (39.1106, 75.1564) (39.9266, 74.3365) (39.9266, 73.3265) (39.9266, 72.3165) (39.1106, 71.4963) (38.1062, 71.4963) knots 0 0 0 0 1 1 1 2 2 2 3 3 3 4 4 4 4
  line L388 (38.1062, 71.4963) -> (37.1015, 71.4963) construction
  line L389 (37.1015, 71.4963) -> (36.2855, 72.3165) construction
  line L390 (36.2855, 72.3165) -> (36.2855, 73.3265) construction
  line L391 (36.2855, 73.3265) -> (36.2855, 74.3365) construction
  line L392 (36.2855, 74.3365) -> (37.1015, 75.1564) construction
  line L393 (37.1015, 75.1564) -> (38.1062, 75.1564) construction
  line L394 (38.1062, 75.1564) -> (39.1106, 75.1564) construction
  line L395 (39.1106, 75.1564) -> (39.9266, 74.3365) construction
  line L396 (39.9266, 74.3365) -> (39.9266, 73.3265) construction
  line L397 (39.9266, 73.3265) -> (39.9266, 72.3165) construction
  line L398 (39.9266, 72.3165) -> (39.1106, 71.4963) construction
  line L399 (39.1106, 71.4963) -> (38.1062, 71.4963) construction
  spline S36 degree 3 poles (38.1062, 55.4975) (37.1015, 55.4975) (36.2855, 56.3174) (36.2855, 57.3274) (36.2855, 58.3377) (37.1015, 59.1576) (38.1062, 59.1576) (39.1106, 59.1576) (39.9266, 58.3377) (39.9266, 57.3274) (39.9266, 56.3174) (39.1106, 55.4975) (38.1062, 55.4975) knots 0 0 0 0 1 1 1 2 2 2 3 3 3 4 4 4 4
  line L400 (38.1062, 55.4975) -> (37.1015, 55.4975) construction
  line L401 (37.1015, 55.4975) -> (36.2855, 56.3174) construction
  line L402 (36.2855, 56.3174) -> (36.2855, 57.3274) construction
  line L403 (36.2855, 57.3274) -> (36.2855, 58.3377) construction
  line L404 (36.2855, 58.3377) -> (37.1015, 59.1576) construction
  line L405 (37.1015, 59.1576) -> (38.1062, 59.1576) construction
  line L406 (38.1062, 59.1576) -> (39.1106, 59.1576) construction
  line L407 (39.1106, 59.1576) -> (39.9266, 58.3377) construction
  line L408 (39.9266, 58.3377) -> (39.9266, 57.3274) construction
  line L409 (39.9266, 57.3274) -> (39.9266, 56.3174) construction
  line L410 (39.9266, 56.3174) -> (39.1106, 55.4975) construction
  line L411 (39.1106, 55.4975) -> (38.1062, 55.4975) construction
  spline S37 degree 3 poles (37.9764, 39.4969) (36.9816, 39.4969) (36.1741, 40.3171) (36.1741, 41.3271) (36.1741, 42.3371) (36.9816, 43.157) (37.9764, 43.157) (38.9716, 43.157) (39.7791, 42.3371) (39.7791, 41.3271) (39.7791, 40.3171) (38.9716, 39.4969) (37.9764, 39.4969) knots 0 0 0 0 1 1 1 2 2 2 3 3 3 4 4 4 4
  line L412 (37.9764, 39.4969) -> (36.9816, 39.4969) construction
  line L413 (36.9816, 39.4969) -> (36.1741, 40.3171) construction
  line L414 (36.1741, 40.3171) -> (36.1741, 41.3271) construction
  line L415 (36.1741, 41.3271) -> (36.1741, 42.3371) construction
  line L416 (36.1741, 42.3371) -> (36.9816, 43.157) construction
  line L417 (36.9816, 43.157) -> (37.9764, 43.157) construction
  line L418 (37.9764, 43.157) -> (38.9716, 43.157) construction
  line L419 (38.9716, 43.157) -> (39.7791, 42.3371) construction
  line L420 (39.7791, 42.3371) -> (39.7791, 41.3271) construction
  line L421 (39.7791, 41.3271) -> (39.7791, 40.3171) construction
  line L422 (39.7791, 40.3171) -> (38.9716, 39.4969) construction
  line L423 (38.9716, 39.4969) -> (37.9764, 39.4969) construction
  spline S38 degree 3 poles (37.9764, 23.4967) (36.9816, 23.4967) (36.1741, 24.3165) (36.1741, 25.3265) (36.1741, 26.3369) (36.9816, 27.1567) (37.9764, 27.1567) (38.9716, 27.1567) (39.7791, 26.3369) (39.7791, 25.3265) (39.7791, 24.3165) (38.9716, 23.4967) (37.9764, 23.4967) knots 0 0 0 0 1 1 1 2 2 2 3 3 3 4 4 4 4
  line L424 (37.9764, 23.4967) -> (36.9816, 23.4967) construction
  line L425 (36.9816, 23.4967) -> (36.1741, 24.3165) construction
  line L426 (36.1741, 24.3165) -> (36.1741, 25.3265) construction
  line L427 (36.1741, 25.3265) -> (36.1741, 26.3369) construction
  line L428 (36.1741, 26.3369) -> (36.9816, 27.1567) construction
  line L429 (36.9816, 27.1567) -> (37.9764, 27.1567) construction
  line L430 (37.9764, 27.1567) -> (38.9716, 27.1567) construction
  line L431 (38.9716, 27.1567) -> (39.7791, 26.3369) construction
  line L432 (39.7791, 26.3369) -> (39.7791, 25.3265) construction
  line L433 (39.7791, 25.3265) -> (39.7791, 24.3165) construction
  line L434 (39.7791, 24.3165) -> (38.9716, 23.4967) construction
  line L435 (38.9716, 23.4967) -> (37.9764, 23.4967) construction
  spline S39 degree 3 poles (37.7824, 7.4961) (36.8024, 7.4961) (36.0058, 8.3163) (36.0058, 9.3263) (36.0058, 10.3363) (36.8024, 11.1562) (37.7824, 11.1562) (38.7606, 11.1562) (39.5572, 10.3363) (39.5572, 9.3263) (39.5572, 8.3163) (38.7606, 7.4961) (37.7824, 7.4961) knots 0 0 0 0 1 1 1 2 2 2 3 3 3 4 4 4 4
  line L436 (37.7824, 7.4961) -> (36.8024, 7.4961) construction
  line L437 (36.8024, 7.4961) -> (36.0058, 8.3163) construction
  line L438 (36.0058, 8.3163) -> (36.0058, 9.3263) construction
  line L439 (36.0058, 9.3263) -> (36.0058, 10.3363) construction
  line L440 (36.0058, 10.3363) -> (36.8024, 11.1562) construction
  line L441 (36.8024, 11.1562) -> (37.7824, 11.1562) construction
  line L442 (37.7824, 11.1562) -> (38.7606, 11.1562) construction
  line L443 (38.7606, 11.1562) -> (39.5572, 10.3363) construction
  line L444 (39.5572, 10.3363) -> (39.5572, 9.3263) construction
  line L445 (39.5572, 9.3263) -> (39.5572, 8.3163) construction
  line L446 (39.5572, 8.3163) -> (38.7606, 7.4961) construction
  line L447 (38.7606, 7.4961) -> (37.7824, 7.4961) construction
  spline S40 degree 3 poles (185.0949, 184.3858) (184.0846, 184.3858) (183.2647, 185.2056) (183.2647, 186.2156) (183.2647, 187.226) (184.0846, 188.0458) (185.0949, 188.0458) (186.105, 188.0458) (186.9248, 187.226) (186.9248, 186.2156) (186.9248, 185.2056) (186.1049, 184.3858) (185.0949, 184.3858) knots 0 0 0 0 1 1 1 2 2 2 3 3 3 4 4 4 4
  line L448 (185.0949, 184.3858) -> (184.0846, 184.3858) construction
  line L449 (184.0846, 184.3858) -> (183.2647, 185.2056) construction
  line L450 (183.2647, 185.2056) -> (183.2647, 186.2156) construction
  line L451 (183.2647, 186.2156) -> (183.2647, 187.226) construction
  line L452 (183.2647, 187.226) -> (184.0846, 188.0458) construction
  line L453 (184.0846, 188.0458) -> (185.0949, 188.0458) construction
  line L454 (185.0949, 188.0458) -> (186.105, 188.0458) construction
  line L455 (186.105, 188.0458) -> (186.9248, 187.226) construction
  line L456 (186.9248, 187.226) -> (186.9248, 186.2156) construction
  line L457 (186.9248, 186.2156) -> (186.9248, 185.2056) construction
  line L458 (186.9248, 185.2056) -> (186.1049, 184.3858) construction
  line L459 (186.1049, 184.3858) -> (185.0949, 184.3858) construction
  spline S41 degree 3 poles (185.0949, 168.3852) (184.0846, 168.3852) (183.2647, 169.2054) (183.2647, 170.2154) (183.2647, 171.2254) (184.0846, 172.0452) (185.0949, 172.0452) (186.105, 172.0452) (186.9248, 171.2254) (186.9248, 170.2154) (186.9248, 169.2054) (186.1049, 168.3852) (185.0949, 168.3852) knots 0 0 0 0 1 1 1 2 2 2 3 3 3 4 4 4 4
  line L460 (185.0949, 168.3852) -> (184.0846, 168.3852) construction
  line L461 (184.0846, 168.3852) -> (183.2647, 169.2054) construction
  line L462 (183.2647, 169.2054) -> (183.2647, 170.2154) construction
  line L463 (183.2647, 170.2154) -> (183.2647, 171.2254) construction
  line L464 (183.2647, 171.2254) -> (184.0846, 172.0452) construction
  line L465 (184.0846, 172.0452) -> (185.0949, 172.0452) construction
  line L466 (185.0949, 172.0452) -> (186.105, 172.0452) construction
  line L467 (186.105, 172.0452) -> (186.9248, 171.2254) construction
  line L468 (186.9248, 171.2254) -> (186.9248, 170.2154) construction
  line L469 (186.9248, 170.2154) -> (186.9248, 169.2054) construction
  line L470 (186.9248, 169.2054) -> (186.1049, 168.3852) construction
  line L471 (186.1049, 168.3852) -> (185.0949, 168.3852) construction
  spline S42 degree 3 poles (185.0314, 156.0436) (184.0267, 156.0436) (183.2111, 155.2237) (183.2111, 154.2137) (183.2111, 153.2034) (184.0267, 152.3835) (185.0314, 152.3835) (186.0362, 152.3835) (186.8532, 153.2034) (186.8532, 154.2137) (186.8532, 155.2237) (186.0362, 156.0436) (185.0314, 156.0436) knots 0 0 0 0 1 1 1 2 2 2 3 3 3 4 4 4 4
  line L472 (185.0314, 156.0436) -> (184.0267, 156.0436) construction
  line L473 (184.0267, 156.0436) -> (183.2111, 155.2237) construction
  line L474 (183.2111, 155.2237) -> (183.2111, 154.2137) construction
  line L475 (183.2111, 154.2137) -> (183.2111, 153.2034) construction
  line L476 (183.2111, 153.2034) -> (184.0267, 152.3835) construction
  line L477 (184.0267, 152.3835) -> (185.0314, 152.3835) construction
  line L478 (185.0314, 152.3835) -> (186.0362, 152.3835) construction
  line L479 (186.0362, 152.3835) -> (186.8532, 153.2034) construction
  line L480 (186.8532, 153.2034) -> (186.8532, 154.2137) construction
  line L481 (186.8532, 154.2137) -> (186.8532, 155.2237) construction
  line L482 (186.8532, 155.2237) -> (186.0362, 156.0436) construction
  line L483 (186.0362, 156.0436) -> (185.0314, 156.0436) construction
  spline S43 degree 3 poles (185.0314, 136.3833) (184.0267, 136.3833) (183.2111, 137.2031) (183.2111, 138.2131) (183.2111, 139.2232) (184.0267, 140.0434) (185.0314, 140.0434) (186.0362, 140.0434) (186.8532, 139.2231) (186.8532, 138.2131) (186.8532, 137.2031) (186.0362, 136.3833) (185.0314, 136.3833) knots 0 0 0 0 1 1 1 2 2 2 3 3 3 4 4 4 4
  line L484 (185.0314, 136.3833) -> (184.0267, 136.3833) construction
  line L485 (184.0267, 136.3833) -> (183.2111, 137.2031) construction
  line L486 (183.2111, 137.2031) -> (183.2111, 138.2131) construction
  line L487 (183.2111, 138.2131) -> (183.2111, 139.2232) construction
  line L488 (183.2111, 139.2232) -> (184.0267, 140.0434) construction
  line L489 (184.0267, 140.0434) -> (185.0314, 140.0434) construction
  line L490 (185.0314, 140.0434) -> (186.0362, 140.0434) construction
  line L491 (186.0362, 140.0434) -> (186.8532, 139.2231) construction
  line L492 (186.8532, 139.2231) -> (186.8532, 138.2131) construction
  line L493 (186.8532, 138.2131) -> (186.8532, 137.2031) construction
  line L494 (186.8532, 137.2031) -> (186.0362, 136.3833) construction
  line L495 (186.0362, 136.3833) -> (185.0314, 136.3833) construction
  spline S44 degree 3 poles (184.902, 120.3827) (183.9068, 120.3827) (183.0993, 121.204) (183.0993, 122.2129) (183.0993, 123.2229) (183.9068, 124.0428) (184.902, 124.0428) (185.8968, 124.0428) (186.7043, 123.2229) (186.7043, 122.2129) (186.7043, 121.204) (185.8968, 120.3827) (184.902, 120.3827) knots 0 0 0 0 1 1 1 2 2 2 3 3 3 4 4 4 4
  line L496 (184.902, 120.3827) -> (183.9068, 120.3827) construction
  line L497 (183.9068, 120.3827) -> (183.0993, 121.204) construction
  line L498 (183.0993, 121.204) -> (183.0993, 122.2129) construction
  line L499 (183.0993, 122.2129) -> (183.0993, 123.2229) construction
  line L500 (183.0993, 123.2229) -> (183.9068, 124.0428) construction
  line L501 (183.9068, 124.0428) -> (184.902, 124.0428) construction
  line L502 (184.902, 124.0428) -> (185.8968, 124.0428) construction
  line L503 (185.8968, 124.0428) -> (186.7043, 123.2229) construction
  line L504 (186.7043, 123.2229) -> (186.7043, 122.2129) construction
  line L505 (186.7043, 122.2129) -> (186.7043, 121.204) construction
  line L506 (186.7043, 121.204) -> (185.8968, 120.3827) construction
  line L507 (185.8968, 120.3827) -> (184.902, 120.3827) construction
  spline S45 degree 3 poles (265.094, 184.3855) (264.084, 184.3855) (263.2642, 185.2058) (263.2642, 186.2158) (263.2642, 187.2258) (264.084, 188.0456) (265.094, 188.0456) (266.104, 188.0456) (266.9242, 187.2258) (266.9242, 186.2158) (266.9242, 185.2058) (266.104, 184.3855) (265.094, 184.3855) knots 0 0 0 0 1 1 1 2 2 2 3 3 3 4 4 4 4
  line L508 (265.094, 184.3855) -> (264.084, 184.3855) construction
  line L509 (264.084, 184.3855) -> (263.2642, 185.2058) construction
  line L510 (263.2642, 185.2058) -> (263.2642, 186.2158) construction
  line L511 (263.2642, 186.2158) -> (263.2642, 187.2258) construction
  line L512 (263.2642, 187.2258) -> (264.084, 188.0456) construction
  line L513 (264.084, 188.0456) -> (265.094, 188.0456) construction
  line L514 (265.094, 188.0456) -> (266.104, 188.0456) construction